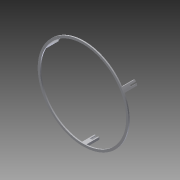
# Autodesk Inventor part: Hallhouder
Saved by Autodesk Inventor 2014 (Build 180170000, 170)
## iProperties
Created: 2015-03-26
Part Number: Hallhouder
Material: ABS Plastic
Document SubType Name: Modeling
Designer: MSI
Density: 1.06 g/cm^3
Appearance: Smooth - White
Author: MSI
Autodesk Inventor part; units mm, degrees
ref_plane "YZ Plane" through (0, 0, 0) normal (1, 0, 0) x (0, 1, 0)
ref_plane "XZ Plane" through (0, 0, 0) normal (0, 1, 0) x (-1, 0, 0)
ref_plane "XY Plane" through (0, 0, 0) normal (0, 0, 1) x (1, 0, 0)
sketch "Sketch1" plane through (0, 0, 0) normal (0, 1, 0) x (-1, 0, 0)
  circle A0 centre (0, 0) radius 39.5
  circle A1 centre (0, 0) radius 37.5
  dimension "d0" = 79
  dimension "d1" = 75
  constraints: 2 centre point, 2 coincident
  measures "d0" diameter of A0
  measures "d1" diameter of A1
extrude "Extrusion1" add sketch "Sketch1" along normal blind 1
sketch "Sketch2" plane through (0, 1, 0) normal (0, 1, 0) x (1, 0, 0)
  circle A0 centre (0, 0) radius 37.5 projected
  circle A1 centre (0, 0) radius 39.5 projected
  line L0 (0, 39.5) -> (0, 37.5) construction
  line L1 (-0.57, 39.24) -> (0, 39.24)
  line L2 (-1.31, 38.5) -> (-1.31, 38.5)
  line L3 (-1.31, 38.5) -> (-1.31, 38.49)
  line L4 (-1.2707, 37.74) -> (0, 37.74)
  line L5 (-0.57, 39.24) -> (-1.31, 38.5)
  line L6 (-1.31, 38.49) -> (-1.2707, 37.74)
  line L7 (0, 0) -> (2.0673, 39.4459) construction
  line L8 (0, 0) -> (-2.0673, 39.4459) construction
  line L9 (1.9626, 37.4486) -> (2.0673, 39.4459)
  line L10 (-1.9626, 37.4486) -> (-2.0673, 39.4459)
  line L11 (-1, 37.74) -> (-1, 37.4867)
  line L12 (0.57, 39.24) -> (0, 39.24)
  line L13 (1.31, 38.5) -> (1.31, 38.5)
  line L14 (1.31, 38.5) -> (1.31, 38.49)
  line L15 (1.2707, 37.74) -> (0, 37.74)
  line L16 (0.57, 39.24) -> (1.31, 38.5)
  line L17 (1.31, 38.49) -> (1.2707, 37.74)
  line L18 (-0.57, 39.24) -> (-0.57, 39.4959)
  line L19 (-0.57, 39.4959) -> (-2.0673, 39.4459)
  line L20 (-1, 37.4867) -> (-1.9646, 37.4867)
  line L21 (0.57, 39.24) -> (0.57, 39.4959)
  line L22 (0.57, 39.4959) -> (2.0673, 39.4459)
  line L23 (1, 37.4867) -> (1, 37.74)
  line L24 (1, 37.4867) -> (1.9646, 37.4867)
  line L25 (-33.6978, -20.1136) -> (-33.9828, -19.62)
  line L26 (-32.687, -20.3845) -> (-32.6783, -20.3795)
  line L27 (-32.0485, -19.9705) -> (-32.6838, -18.87)
  line L28 (-33.6978, -20.1136) -> (-32.687, -20.3845)
  line L29 (-32.6783, -20.3795) -> (-32.0485, -19.9705)
  line L30 (0, 0) -> (-33.1275, -21.5132) construction
  line L31 (-33.4127, -17.0246) -> (-35.1948, -17.9326)
  line L32 (-31.4501, -20.424) -> (-33.1275, -21.5132)
  line L33 (-32.1838, -19.736) -> (-31.9644, -19.6094)
  line L34 (-33.9883, -18.1105) -> (-33.3191, -17.7695)
  line L35 (-33.3191, -17.7695) -> (-32.6838, -18.87)
  line L36 (-34.2678, -19.1264) -> (-33.997, -18.1155)
  line L37 (-34.2678, -19.1264) -> (-33.9828, -19.62)
  line L38 (-33.997, -18.1155) -> (-33.9883, -18.1105)
  line L39 (-33.6978, -20.1136) -> (-33.9194, -20.2416)
  line L40 (-33.9194, -20.2416) -> (-33.1275, -21.5132)
  line L41 (-31.9644, -19.6094) -> (-31.4821, -20.4447)
  line L42 (-34.2678, -19.1264) -> (-34.4894, -19.2543)
  line L43 (-34.4894, -19.2543) -> (-35.1948, -17.9326)
  line L44 (-32.9644, -17.8773) -> (-33.1838, -18.004)
  line L45 (-32.9644, -17.8773) -> (-33.4467, -17.0419)
  line L46 (34.2678, -19.1264) -> (33.9828, -19.62)
  line L47 (33.997, -18.1155) -> (33.9883, -18.1105)
  line L48 (33.3191, -17.7695) -> (32.6838, -18.87)
  line L49 (34.2678, -19.1264) -> (33.997, -18.1155)
  line L50 (33.9883, -18.1105) -> (33.3191, -17.7695)
  line L51 (0, 0) -> (35.1948, -17.9326) construction
  line L52 (31.4501, -20.424) -> (33.1275, -21.5132)
  line L53 (33.4127, -17.0246) -> (35.1948, -17.9326)
  line L54 (33.1838, -18.004) -> (32.9644, -17.8773)
  line L55 (32.6783, -20.3795) -> (32.0485, -19.9705)
  line L56 (32.0485, -19.9705) -> (32.6838, -18.87)
  line L57 (33.6978, -20.1136) -> (32.687, -20.3845)
  line L58 (33.6978, -20.1136) -> (33.9828, -19.62)
  line L59 (32.687, -20.3845) -> (32.6783, -20.3795)
  line L60 (34.2678, -19.1264) -> (34.4894, -19.2543)
  line L61 (34.4894, -19.2543) -> (35.1948, -17.9326)
  line L62 (32.9644, -17.8773) -> (33.4467, -17.0419)
  line L63 (33.6978, -20.1136) -> (33.9194, -20.2416)
  line L64 (33.9194, -20.2416) -> (33.1275, -21.5132)
  line L65 (31.9644, -19.6094) -> (32.1838, -19.736)
  line L66 (31.9644, -19.6094) -> (31.4821, -20.4447)
  line L67 (-33.1838, -18.004) -> (-33.3191, -17.7695)
  line L68 (-33.3191, -17.7695) -> (-33.9883, -18.1105)
  line L69 (-33.997, -18.1155) -> (-33.9883, -18.1105)
  line L70 (-34.2678, -19.1264) -> (-33.997, -18.1155)
  line L71 (-33.6978, -20.1136) -> (-32.687, -20.3845)
  line L72 (-32.0485, -19.9705) -> (-32.6783, -20.3795)
  line L73 (-32.0485, -19.9705) -> (-32.1838, -19.736)
  line L74 (34.2678, -19.1264) -> (33.997, -18.1155)
  line L75 (33.1838, -18.004) -> (33.3191, -17.7695)
  line L76 (33.6978, -20.1136) -> (32.687, -20.3845)
  point P0 (-1.31, 39.24)
  point P1 (-1.31, 37.74)
  point P2 (0, 38.5)
  point P3 (1.31, 37.74)
  point P4 (-33.3278, -20.7545)
  point P5 (-32.0288, -20.0045)
  point P6 (-33.3388, -17.7355)
  point P7 (34.6378, -18.4855)
  point P8 (33.3388, -17.7355)
  point P9 (32.0288, -20.0045)
  dimension "d4" = 1.31
  dimension "d5" = 0.74
  dimension "d6" = 0.76
  dimension "d7" = 0.74
  dimension "d8" = 45
  dimension "d9" = 0.75
  dimension "d10" = 3
  dimension "d11" = 3
  dimension "d12" = 1
  dimension "d15" = 360
  constraints: 154 end point, 33 point on line, 9 symmetric about line, 7 collinear, 7 point on circle, 6 perpendicular, 2 parallel, 2 vertical alignment, 1 horizontal alignment, 1 midpoint, 1 vertical, 148 other
  measures "d4" distance of point (-1.31, 39.24) L1.end
  measures "d5" distance of point (-1.31, 39.24) L2.end
  measures "d6" distance of L2.end point (-1.31, 37.74)
  measures "d7" distance of L1.start point (-1.31, 39.24)
  measures "d8" angle of L1 L5
  measures "d9" distance of L3.end point (-1.31, 37.74)
  measures "d10" angle of L3 L6
  measures "d11" angle of L7 L0
  measures "d12" distance between parallel lines of L0 L11
extrude "Extrusion2" add sketch "Sketch2" along normal blind 11 contours L23 L15 L17 L14 L16 L21 L22 L9 L24 | L62 L53 L61 L60 L49 L47 L50 L48 L54 | L20 L10 L19 L18 L5 L3 L6 L4 L11 | L65 L56 L55 L59 L57 L63 L64 L52 L66 | L44 L35 L34 L38 L36 L42 L43 L31 L45 | L41 L32 L40 L39 L28 L26 L29 L27 L33
sketch "Sketch3" plane through (0, 1, 0) normal (0, 1, 0) x (1, 0, 0)
  line L0 (33.1838, -18.004) -> (32.9644, -17.8773) projected
  arc A0 (31.9644, -19.6094) -> (32.9644, -17.8773) centre (0, 0) ccw projected
  line L1 (31.9644, -19.6094) -> (32.1838, -19.736) projected
  line L2 (32.1838, -19.736) -> (32.0485, -19.9705) projected
  line L3 (32.0485, -19.9705) -> (32.6783, -20.3795) projected
  line L4 (32.6783, -20.3795) -> (32.687, -20.3845) projected
  line L5 (32.687, -20.3845) -> (33.6978, -20.1136) projected
  line L6 (33.6978, -20.1136) -> (33.9194, -20.2416) projected
  arc A1 (33.9194, -20.2416) -> (34.4894, -19.2543) centre (0, 0) ccw projected
  line L7 (34.4894, -19.2543) -> (34.2678, -19.1264) projected
  line L8 (34.2678, -19.1264) -> (33.997, -18.1155) projected
  line L9 (33.997, -18.1155) -> (33.9883, -18.1105) projected
  line L10 (33.9883, -18.1105) -> (33.3191, -17.7695) projected
  line L11 (33.3191, -17.7695) -> (33.1838, -18.004) projected
extrude "Extrusion3" add sketch "Sketch3" along normal blind 6
sketch "Sketch4" plane through (0, 1, 0) normal (0, 1, 0) x (1, 0, 0)
  line L0 (-32.1838, -19.736) -> (-31.9644, -19.6094) projected
  arc A0 (-32.9644, -17.8773) -> (-31.9644, -19.6094) centre (0, 0) ccw projected
  line L1 (-32.9644, -17.8773) -> (-33.1838, -18.004) projected
  line L2 (-33.1838, -18.004) -> (-33.3191, -17.7695) projected
  line L3 (-33.3191, -17.7695) -> (-33.9883, -18.1105) projected
  line L4 (-33.9883, -18.1105) -> (-33.997, -18.1155) projected
  line L5 (-33.997, -18.1155) -> (-34.2678, -19.1264) projected
  line L6 (-34.2678, -19.1264) -> (-34.4894, -19.2543) projected
  arc A1 (-34.4894, -19.2543) -> (-33.9194, -20.2416) centre (0, 0) ccw projected
  line L7 (-33.9194, -20.2416) -> (-33.6978, -20.1136) projected
  line L8 (-33.6978, -20.1136) -> (-32.687, -20.3845) projected
  line L9 (-32.687, -20.3845) -> (-32.6783, -20.3795) projected
  line L10 (-32.6783, -20.3795) -> (-32.0485, -19.9705) projected
  line L11 (-32.0485, -19.9705) -> (-32.1838, -19.736) projected
extrude "Extrusion4" add sketch "Sketch4" along normal blind 6
sketch "Sketch5" plane through (0, 1, 0) normal (0, 1, 0) x (1, 0, 0)
  line L0 (-0.57, 39.4959) -> (-0.57, 39.24) projected
  line L1 (-0.57, 39.24) -> (-1.31, 38.5) projected
  line L2 (-1.31, 38.5) -> (-1.31, 38.49) projected
  line L3 (-1.31, 38.49) -> (-1.2707, 37.74) projected
  line L4 (-1.2707, 37.74) -> (-1, 37.74) projected
  line L5 (-1, 37.74) -> (-1, 37.4867) projected
  arc A0 (1, 37.4867) -> (-1, 37.4867) centre (0, 0) ccw projected
  line L6 (1, 37.4867) -> (1, 37.74) projected
  line L7 (1, 37.74) -> (1.2707, 37.74) projected
  line L8 (1.2707, 37.74) -> (1.31, 38.49) projected
  line L9 (1.31, 38.49) -> (1.31, 38.5) projected
  line L10 (1.31, 38.5) -> (0.57, 39.24) projected
  line L11 (0.57, 39.24) -> (0.57, 39.4959) projected
  arc A1 (0.57, 39.4959) -> (-0.57, 39.4959) centre (0, 0) ccw projected
extrude "Extrusion5" add sketch "Sketch5" along normal blind 6
body "Solid1"
